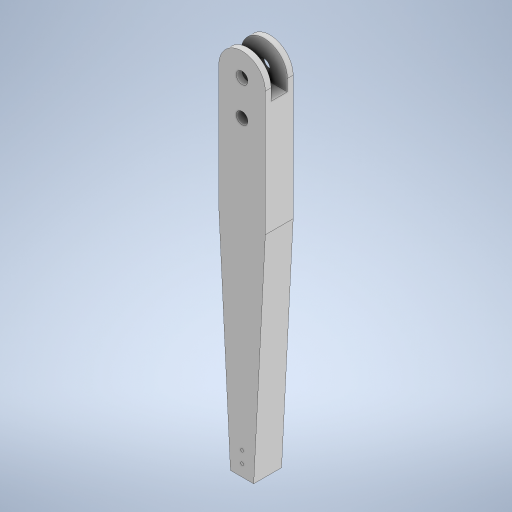
# Autodesk Inventor part: legparts_06(three)
Saved by Autodesk Inventor 2024.3 (Build 283343000, 343)
## iProperties
Created: 2024-10-20
Part Number: legparts_06(three)
Material: 一般
Document SubType Name: Modeling
Designer: 佐藤智貴
Density: 1 g/cm^3
Appearance: 既定
Mass: 239.731 g
Surface Area: 419.569 cm^2
Volume: 239.731 cm^3
Author: 佐藤智貴
Autodesk Inventor part; units mm, degrees
ref_plane "YZ Plane" through (0, 0, 0) normal (1, 0, 0) x (0, 1, 0)
ref_plane "XZ Plane" through (0, 0, 0) normal (0, 1, 0) x (-1, 0, 0)
ref_plane "XY Plane" through (0, 0, 0) normal (0, 0, 1) x (1, 0, 0)
sketch "スケッチ1" plane through (0, 0, 0) normal (0, 0, 1) x (1, 0, 0)
  line L0 (0, 0) -> (40, 0)
  line L1 (40, 0) -> (40, 318)
  line L2 (40, 318) -> (0, 318)
  line L3 (0, 318) -> (0, 0)
  line L4 (10, 0) -> (0, 190.8114)
  line L5 (40, 190.8114) -> (30, 0)
  dimension "d0" = 40
  dimension "d1" = 318
  dimension "d64" = 20
  dimension "d65" = 10
  dimension "d66" = 87
  dimension "d67" = 87
  constraints: 12 end point, 4 point on line, 2 parallel, 1 horizontal, 1 perpendicular
  measures "d0" distance of L1.end L2.end
  measures "d1" distance of L0.end L1.end
  measures "d64" distance of L5.end L4.start
  measures "d65" distance of L0.start L4.start
  measures "d66" angle of L0 L4
  measures "d67" angle of L0 L5
extrude "押し出し1" add sketch "スケッチ1" along normal blind 24 contours L4 L3 L2 L1 L5 L0
sketch "スケッチ6" plane through (0, 0, 24) normal (0, 0, 1) x (1, 0, 0)
  circle A0 centre (20, 268) radius 5
  line L0 (40, 318) -> (0, 318) projected
  line L1 (40, 190.8114) -> (40, 318) projected
  circle A1 centre (20, 20) radius 1.2295
  circle A2 centre (20, 10) radius 1.2295
  line L2 (0, 0) -> (30, 0) projected
  circle A3 centre (20, 298) radius 5
  point P0 (20, 318)
  point P1 (40, 0)
  dimension "d42" = 10
  dimension "d44" = 20
  dimension "d45" = 2.459
  dimension "d46" = 2.459
  dimension "d47" = 10
  dimension "d48" = 10
  dimension "d49" = 20
  dimension "d50" = 20
  dimension "d53" = 10
  dimension "d54" = 20
  dimension "d55" = 30
  dimension "d56" = 20
  constraints: 4 centre point, 1 midpoint
  measures "d42" diameter of A0
  measures "d44" distance from line of L1 A0.centre
  measures "d45" diameter of A1
  measures "d46" diameter of A2
  measures "d47" distance from line of L2 A2.centre
  measures "d48" distance of A2.centre A1.centre
  measures "d49" distance from line of L1 A2.centre
  measures "d50" distance from line of L1 A1.centre
  measures "d53" diameter of A3
  measures "d54" distance from line of L0 A3.centre
  measures "d55" distance of A3.centre A0.centre
  measures "d56" distance from line of L1 A3.centre
extrude "押し出し4" cut sketch "スケッチ6" against normal through all
sketch "スケッチ8" plane through (0, 0, 0) normal (-1, 0, 0) x (0, 0, 1)
  line L0 (0, 318) -> (24, 318) projected
  line L1 (5, 318) -> (19, 318)
  line L2 (19, 318) -> (19, 288)
  line L3 (19, 288) -> (5, 288)
  line L4 (5, 288) -> (5, 318)
  line L5 (0, 318) -> (0, 0) projected
  dimension "d57" = 5
  dimension "d58" = 14
  dimension "d59" = 30
  constraints: 8 end point, 2 parallel, 1 horizontal, 1 perpendicular, 1 point on line
  measures "d57" distance between parallel lines of L5 L4
  measures "d58" distance between parallel lines of L4 L2
  measures "d59" distance between parallel lines of L0 L3
extrude "押し出し5" cut sketch "スケッチ8" against normal through all
fillet "フィレット1" radius 20 4 edges at (40, 318, 21.5) (40, 318, 2.5) (0, 318, 2.5) (0, 318, 21.5)
equation "\"d67\" = d66"
equation "\"d45\" = d46"
equation "\"d48\" = d47"
equation "\"d50\" = d49"
